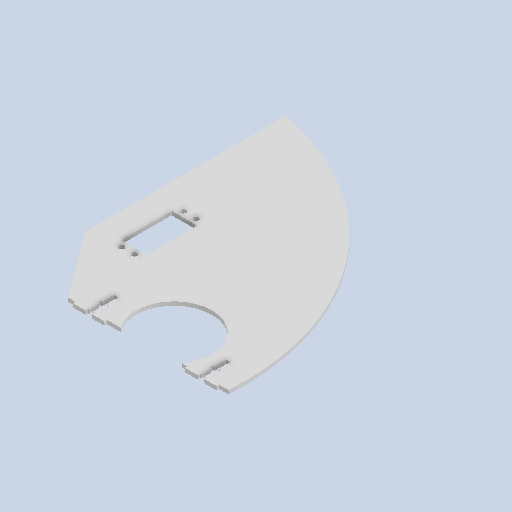
# Autodesk Inventor part: боковые стороны головы
Saved by Autodesk Inventor 2023.2 (Build 272271030, 271C)
## iProperties
Created: 2024-01-31
Part Number: боковые стороны головы
Material: Типовые
Document SubType Name: Modeling
Designer: I9232
Density: 1 g/cm^3
Appearance: По умолчанию
Author: I9232
Autodesk Inventor part; units mm, degrees
ref_plane "YZ Plane" through (0, 0, 0) normal (1, 0, 0) x (0, 1, 0)
ref_plane "XZ Plane" through (0, 0, 0) normal (0, 1, 0) x (-1, 0, 0)
ref_plane "XY Plane" through (0, 0, 0) normal (0, 0, 1) x (1, 0, 0)
sketch "Эскиз1" plane through (0, 0, 0) normal (0, 1, 0) x (-1, 0, 0)
  line L0 (-165, -96.7538) -> (-38.405, -96.7538)
  line L1 (0, -148.7467) -> (0, -306.7538)
  arc A0 (-165, -96.7538) -> (0, -306.7538) centre (36.5744, -108.1954) ccw
  line L2 (-38.405, -96.7538) -> (0, -148.7467)
  point P0 (0, 0)
  point P1 (-167.673, -110.7197)
  constraints: 6 end point, 2 point on circle, 1 centre point, 1 horizontal, 1 perpendicular
extrude "Выдавливание2" add sketch "Эскиз1" along normal blind 3
sketch "Эскиз3" plane through (0, 0, 0) normal (0, -1, 0) x (1, 0, 0)
  circle A0 centre (103.9785, -114.6678) radius 30
  point P0 (0, 0)
  dimension "d4" = 60
  constraints: 1 centre point
  measures "d4" diameter of A0
extrude "Выдавливание3" cut sketch "Эскиз3" against normal through all
sketch "Эскиз4" plane through (0, 3, 0) normal (0, 1, 0) x (1, 0, 0)
  line L0 (40.1, 196.7538) -> (20, 196.7538)
  line L1 (20, 196.7538) -> (20, 156.7538)
  line L2 (20, 156.7538) -> (40.1, 156.7538)
  line L3 (40.1, 156.7538) -> (40.1, 196.7538)
  line L4 (40.1, 156.7538) -> (40.1, 149.7538) construction
  line L5 (40.1, 149.7538) -> (30.05, 149.7538) construction
  line L6 (20, 149.7538) -> (20, 156.7538) construction
  line L7 (40.1, 196.7538) -> (40.1, 203.7538) construction
  line L8 (40.1, 203.7538) -> (20, 203.7538) construction
  line L9 (20, 203.7538) -> (20, 196.7538) construction
  line L10 (30.05, 203.7538) -> (30.05, 196.7538) construction
  line L11 (30.05, 156.7538) -> (30.05, 149.7538) construction
  line L12 (30.05, 149.7538) -> (20, 149.7538) construction
  line L13 (35.075, 149.7538) -> (35.075, 156.7538) construction
  line L14 (25.025, 149.7538) -> (25.025, 156.7538) construction
  circle A0 centre (35.075, 152.4038) radius 2.15
  circle A1 centre (25.025, 152.4038) radius 2.15
  line L15 (40.1, 176.7538) -> (20, 176.7538) construction
  circle A2 centre (35.075, 201.1038) radius 2.15
  circle A3 centre (25.025, 201.1038) radius 2.15
  line L16 (0, 306.7538) -> (0, 148.7467) projected
  line L17 (35.075, 201.1038) -> (35.075, 196.7538) construction
  line L18 (25.025, 201.1038) -> (25.025, 196.7538) construction
  line L19 (0, 96.7538) -> (79.9142, 96.7538) projected
  point P0 (0, 0)
  dimension "d9" = 20.1
  dimension "d10" = 40
  dimension "d11" = 7
  dimension "d12" = 7
  dimension "d13" = 4.3
  dimension "d14" = 4.3
  dimension "d15" = 4.35
  dimension "d16" = 4.35
  dimension "d37" = 20
  dimension "d38" = 60
  constraints: 36 end point, 11 perpendicular, 7 midpoint, 6 point on line, 4 centre point, 2 parallel, 2 symmetric about line, 1 horizontal, 1 vertical, 2 other
  measures "d9" distance of L1.end L2.end
  measures "d10" distance of L0.end L1.end
  measures "d11" distance of L2.end L4.end
  measures "d12" distance of L0.start L7.end
  measures "d13" diameter of A0
  measures "d14" diameter of A1
  measures "d15" distance of L13.end A0.centre
  measures "d16" distance of A1.centre L14.end
  measures "d37" distance between parallel lines of L16 L1
  measures "d38" distance from line of L19 L11.start
extrude "Выдавливание4" cut sketch "Эскиз4" against normal blind 10
sketch "Эскиз6" plane through (165, 0, -96.7538) normal (0, 0, 1) x (1, 0, 0)
  line L0 (-36.9572, 3) -> (0, 3) construction
  line L1 (-7.5115, 3) -> (-17.5115, 3)
  line L2 (-17.5115, 3) -> (-17.5115, 0)
  line L3 (-17.5115, 0) -> (-7.5115, 0)
  line L4 (-7.5115, 0) -> (-7.5115, 3)
  line L5 (-22.5115, 3) -> (-32.5115, 3)
  line L6 (-32.5115, 3) -> (-32.5115, 0)
  line L7 (-32.5115, 0) -> (-22.5115, 0)
  line L8 (-22.5115, 0) -> (-22.5115, 3)
  line L9 (-96.0168, 3) -> (-106.0168, 3)
  line L10 (-106.0168, 3) -> (-106.0168, 0)
  line L11 (-106.0168, 0) -> (-96.0168, 0)
  line L12 (-96.0168, 0) -> (-96.0168, 3)
  line L13 (-111.0168, 3) -> (-121.0168, 3)
  line L14 (-121.0168, 3) -> (-121.0168, 0)
  line L15 (-121.0168, 0) -> (-111.0168, 0)
  line L16 (-111.0168, 0) -> (-111.0168, 3)
  line L17 (-165, 0) -> (-85.0858, 0) projected
  point P0 (0, 0)
  point P1 (-22.5115, 1.5)
  point P2 (-17.5115, 1.5)
  point P3 (-122.3404, 3.4597)
  point P4 (-111.0168, 1.5)
  point P5 (-106.0168, 1.5)
  point P6 (-101.0168, 0)
  point P7 (-116.0168, 0)
  dimension "d20" = 10
  dimension "d21" = 10
  dimension "d22" = 3
  dimension "d23" = 5
  dimension "d24" = 10
  dimension "d25" = 10
  dimension "d26" = 3
  dimension "d27" = 5
  dimension "d28" = 3
  constraints: 32 end point, 8 parallel, 6 midpoint, 4 horizontal, 4 perpendicular, 4 point on line
  measures "d20" distance of L2.end L3.end
  measures "d21" distance of L6.end L7.end
  measures "d22" distance of L7.end L5.start
  measures "d23" distance of point (-22.511, 1.5) point (-17.511, 1.5)
  measures "d24" distance of L10.end L11.end
  measures "d25" distance of L14.end L15.end
  measures "d26" distance of L15.end L13.start
  measures "d27" distance of point (-111.017, 1.5) point (-106.017, 1.5)
  measures "d28" distance of L11.end L9.start
extrude "Выдавливание5" add sketch "Эскиз6" along normal blind 2
sketch "Эскиз7" plane through (0, 0, 0) normal (0, -1, 0) x (1, 0, 0)
  line L0 (53.9832, -96.7538) -> (58.9832, -96.7538) projected
  line L1 (58.9832, -96.7538) -> (53.9832, -96.7538)
  line L2 (56.4832, -96.7538) -> (58.2332, -96.7538)
  line L3 (58.2332, -116.7538) -> (56.4832, -116.7538)
  line L4 (56.4832, -116.7538) -> (56.4832, -96.7538) construction
  line L5 (54.7332, -116.7538) -> (56.4832, -116.7538)
  line L6 (53.4332, -104.8538) -> (53.4332, -107.3538)
  line L7 (59.5332, -107.3538) -> (59.5332, -104.8538)
  line L8 (59.5332, -104.8538) -> (53.4332, -107.3538) construction
  line L9 (53.4332, -104.8538) -> (59.5332, -107.3538) construction
  line L10 (56.4832, -104.8538) -> (56.4832, -106.1038)
  line L11 (143.0775, -96.7538) -> (146.8996, -96.7538)
  line L12 (146.8996, -96.7538) -> (143.0775, -96.7538)
  line L13 (144.9885, -96.7538) -> (146.7385, -96.7538)
  line L14 (146.7385, -116.7538) -> (144.9885, -116.7538)
  line L15 (144.9885, -116.7538) -> (144.9885, -96.7538) construction
  line L16 (143.2385, -116.7538) -> (144.9885, -116.7538)
  line L17 (141.9385, -104.8538) -> (141.9385, -107.3538)
  line L18 (148.0385, -107.3538) -> (148.0385, -104.8538)
  line L19 (148.0385, -104.8538) -> (141.9385, -107.3538) construction
  line L20 (141.9385, -104.8538) -> (148.0385, -107.3538) construction
  line L21 (144.9885, -104.8538) -> (144.9885, -106.1038)
  line L22 (142.4885, -96.7538) -> (147.4885, -96.7538) projected
  line L23 (148.0385, -104.8538) -> (146.7385, -104.8538)
  line L24 (143.2385, -104.8538) -> (141.9385, -104.8538)
  line L25 (146.7385, -96.7538) -> (146.7385, -104.8538)
  line L26 (146.7385, -107.3538) -> (146.7385, -116.7538)
  line L27 (141.9385, -107.3538) -> (143.2385, -107.3538)
  line L28 (146.7385, -107.3538) -> (148.0385, -107.3538)
  line L29 (143.2385, -96.7538) -> (143.2385, -104.8538)
  line L30 (143.2385, -107.3538) -> (143.2385, -116.7538)
  line L31 (59.5332, -104.8538) -> (58.2332, -104.8538)
  line L32 (54.7332, -104.8538) -> (53.4332, -104.8538)
  line L33 (53.4332, -107.3538) -> (54.7332, -107.3538)
  line L34 (58.2332, -107.3538) -> (59.5332, -107.3538)
  line L35 (58.2332, -96.7538) -> (58.2332, -104.8538)
  line L36 (58.2332, -107.3538) -> (58.2332, -116.7538)
  line L37 (54.7332, -96.7538) -> (54.7332, -104.8538)
  line L38 (54.7332, -107.3538) -> (54.7332, -116.7538)
  point P0 (0, 0)
  dimension "d31" = 20
  dimension "d32" = 3.5
  dimension "d33" = 6.1
  dimension "d34" = 2.5
  dimension "d43" = 8.1
  dimension "d44" = 20
  dimension "d45" = 3.5
  dimension "d46" = 6.1
  dimension "d47" = 2.5
  dimension "d48" = 8.1
  constraints: 74 end point, 16 parallel, 10 perpendicular, 7 midpoint, 6 horizontal, 4 collinear, 4 symmetric about line, 1 point on line
  measures "d31" distance of L2.end L3.start
  measures "d32" distance of L5.start L3.start
  measures "d33" distance of L6.end L7.start
  measures "d34" distance of L6.start L6.end
  measures "d43" distance of point (56.483, -96.754) L10.start
  measures "d44" distance of L13.end L14.start
  measures "d45" distance of L16.start L14.start
  measures "d46" distance of L17.end L18.start
  measures "d47" distance of L17.start L17.end
  measures "d48" distance of L21.start point (144.989, -96.754)
extrude "Выдавливание6" cut sketch "Эскиз7" against normal blind 3
